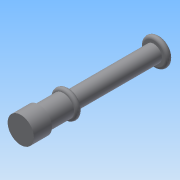
# Autodesk Inventor part: hand
Saved by Autodesk Inventor 2014 (Build 180170000, 170)
## iProperties
Created: 2018-01-03
Part Number: hand
Material: 一般
Document SubType Name: Modeling
Designer: user
Density: 1 g/cm^3
Appearance: 預設
Author: user
Autodesk Inventor part; units mm, degrees
ref_plane "YZ Plane" through (0, 0, 0) normal (1, 0, 0) x (0, 1, 0)
ref_plane "XZ Plane" through (0, 0, 0) normal (0, 1, 0) x (-1, 0, 0)
ref_plane "XY Plane" through (0, 0, 0) normal (0, 0, 1) x (1, 0, 0)
sketch "草圖1" plane through (0, 0, 0) normal (0, 0, 1) x (1, 0, 0)
  circle A0 centre (0, 0) radius 7.25
  dimension "d0" = 14.5
  constraints: 1 centre point, 1 coincident
  measures "d0" diameter of A0
extrude "擠出1" add sketch "草圖1" along normal blind 10
sketch "草圖2" plane through (0, 0, 0) normal (0, 0, -1) x (-1, 0, 0)
  circle A0 centre (0, 0) radius 7.25 construction
  circle A1 centre (0, 0) radius 6
  dimension "d3" = 12
  constraints: 1 centre point, 1 coincident
  measures "d3" diameter of A1
extrude "擠出2" add sketch "草圖2" along normal blind 15
sketch "草圖3" plane through (0, 0, 0) normal (1, 0, 0) x (0, 1, 0)
  line L0 (-6, -15) -> (6, -15) construction
  circle A0 centre (6, -15) radius 1.5
  line L1 (0, -27.8) -> (0, 16.3) projected
  point P0 (0, 0)
  dimension "d6" = 3
  constraints: 1 centre point, 1 coincident
  measures "d6" diameter of A0
revolve "迴轉1" add sketch "草圖3" angle 360 about axis through (0, 0, -10) along (0, 0, 1)
sketch "草圖4" plane through (0, 0, -15) normal (0, 0, -1) x (-1, 0, 0)
  circle A0 centre (0, 0) radius 4.5 projected
extrude "擠出3" add sketch "草圖4" along normal blind 50
sketch "草圖9" plane through (0, 0, 0) normal (1, 0, 0) x (0, 1, 0)
  arc A0 (6, -16.5) -> (6, -13.5) centre (6, -15) ccw construction
  line L0 (6, -15) -> (6, -68.4054) construction
  line L1 (-4.5, -65) -> (4.5, -65) construction
  line L2 (0, -65) -> (6, -65) construction
  arc A1 (6, -66.5) -> (6, -63.5) centre (6, -65) ccw
  line L3 (0, -84.0865) -> (0, 25.6811) projected
  line L4 (6, -66.5) -> (0, -66.5)
  line L5 (0, -65) -> (4.5, -65) construction
  line L6 (6, -63.5) -> (0, -63.5)
  line L7 (0, -66.5) -> (0, -63.5)
  point P0 (0, 0)
  dimension "d14" = 3
  constraints: 12 end point, 5 point on line, 2 collinear, 2 perpendicular, 2 point on circle, 2 tangent, 1 centre point, 1 coincident, 1 midpoint, 1 vertical
  measures "d14" diameter of A1
revolve "迴轉2" add sketch "草圖9" angle 360 about axis through (0, 0, -10) along (0, 0, 1)
